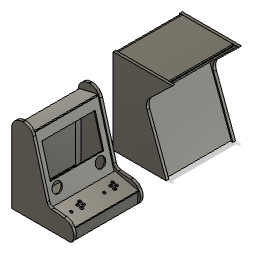
Curvy-Cab (Autodesk Fusion 360 design; units mm, degrees)
Autodesk Fusion 360 part; units mm, degrees
note: some values were not read from the file. Chosen so that the rebuilt part matches the saved one: which bodies a step acts on; which face or edge a step refers to; a side. Set by a fixed rule: which sketch regions a step uses.
sketch "Sketch1" plane through (0, 0, 0) normal (0, 0, 1) x (1, 0, 0)
  line L0 (0, 0) -> (508, 0)
  line L1 (0, 0) -> (0, 1478.2685)
  line L2 (205.4071, 1505.406) -> (336.1627, 1032.1467)
  line L3 (381.7704, 993.9985) -> (500.0828, 983.0939)
  line L4 (561.4783, 808.976) -> (349.2633, 603.2383)
  line L5 (324.7055, 495.0118) -> (508, 0)
  arc A0 (336.1627, 1032.1467) -> (381.7704, 993.9985) centre (386.57, 1046.0736) ccw
  arc A1 (561.4783, 808.976) -> (500.0828, 983.0939) centre (490.7581, 881.9227) ccw
  arc A2 (349.2633, 603.2383) -> (324.7055, 495.0118) centre (419.9835, 530.2916) ccw
  line L6 (100.21, 1579.8589) -> (106.0861, 1579.9393)
  arc A3 (100.21, 1579.8589) -> (0, 1478.2685) centre (101.6, 1478.2685) ccw
  arc A4 (205.4071, 1505.406) -> (106.0861, 1579.9393) centre (107.4762, 1478.3489) ccw
  point P0 (0, 1651)
  dimension "d1" = 508
  dimension "d2" = 1651
  dimension "d48" = 101.6
  dimension "d49" = 101.6
  constraint coincident L0.start L1.start
  constraint horizontal L0
  constraint perpendicular L0 L1
  constraint coincident P0 L1
  constraint tangent L2 A0
  constraint tangent L3 A0
  constraint tangent L3 A1
  constraint tangent L4 A1
  constraint tangent L4 A2
  constraint tangent L5 A2
  constraint tangent L1 A3
  constraint tangent L6 A3
  constraint tangent L2 A4
  constraint tangent L6 A4
  measures "d1" distance of L0.start L0.end
  measures "d2" distance of L0.start P0
  measures "d48" radius of A3
  measures "d49" radius of A4
extrude "Extrude1" add sketch "Sketch1" along normal blind 25.4 makes body 1
copy_body "CopyPasteBodies2" bodies 1 makes body 2
move_body "Move5" bodies 2 to x (1, 0, 0) y (0, 1, 0) z (0, 0, 1) at (0, 0, -635)
sketch "Sketch17" plane through (0, 0, 0) normal (0, 0, 1) x (1, 0, 0)
  line L0 (0, 0) -> (502.8778, 0)
  constraint coincident L0.start origin
  constraint horizontal L0
extrude "Extrude15" add sketch "Sketch17" against normal up to surface (609.6 mm away) thin wall 12.7 on the left separate body open curves L0 makes body 3
extrude "Extrude16" cut 1 faces at (0, 8.4667, -203.2) along direction (1, 0, 0) blind 25.4 on bodies 3 bodies 3
extrude "Extrude17" cut 1 faces at (502.8778, 8.4667, -203.2) along direction (-1, 0, 0) blind 25.4 on bodies 3 bodies 3
sketch "Sketch19" plane through (0, 0, 0) normal (0, 0, -1) x (-1, 0, 0)
  line L0 (-205.4071, 1505.406) -> (-336.1627, 1032.1467)
  arc A0 (-381.7704, 993.9985) -> (-336.1627, 1032.1467) centre (-386.57, 1046.0736) ccw
  line L1 (-381.7704, 993.9985) -> (-500.0828, 983.0939)
  arc A1 (-500.0828, 983.0939) -> (-561.4783, 808.976) centre (-490.7581, 881.9227) ccw
  line L2 (-561.4783, 808.976) -> (-349.2633, 603.2383)
  arc A2 (-324.7055, 495.0118) -> (-349.2633, 603.2383) centre (-419.9835, 530.2916) ccw
  line L3 (-324.7055, 495.0118) -> (-508, 0)
  line L4 (-508, 0) -> (0, 0)
  line L5 (0, 0) -> (0, 1478.2685)
  arc A3 (0, 1478.2685) -> (-100.21, 1579.8589) centre (-101.6, 1478.2685) ccw
  line L6 (-100.21, 1579.8589) -> (-106.0861, 1579.9393)
  arc A4 (-106.0861, 1579.9393) -> (-205.4071, 1505.406) centre (-107.4762, 1478.3489) ccw
  line L7 (0, 0) -> (0, 1478.2685)
  constraint coincident L4.end L5.start
  constraint coincident L5.end A3.start
extrude "Extrude18" add sketch "Sketch19" along normal up to surface (609.6 mm away) thin wall 12.7 on the left separate body open curves L7 makes body 4
move_body "Move6" bodies 4 to x (1, 0, 0) y (0, 1, 0) z (0, 0, 1) at (12.7, 0, 0)
sketch "Sketch20" plane through (0, 0, 0) normal (0, 0, -1) x (-1, 0, 0)
  line L0 (-205.4071, 1505.406) -> (-336.1627, 1032.1467)
  arc A0 (-381.7704, 993.9985) -> (-336.1627, 1032.1467) centre (-386.57, 1046.0736) ccw
  line L1 (-381.7704, 993.9985) -> (-500.0828, 983.0939)
  arc A1 (-500.0828, 983.0939) -> (-561.4783, 808.976) centre (-490.7581, 881.9227) ccw
  line L2 (-561.4783, 808.976) -> (-349.2633, 603.2383)
  arc A2 (-324.7055, 495.0118) -> (-349.2633, 603.2383) centre (-419.9835, 530.2916) ccw
  line L3 (-324.7055, 495.0118) -> (-508, 0)
  line L4 (-508, 0) -> (0, 0)
  line L5 (0, 0) -> (0, 1478.2685)
  arc A3 (0, 1478.2685) -> (-100.21, 1579.8589) centre (-101.6, 1478.2685) ccw
  line L6 (-100.21, 1579.8589) -> (-106.0861, 1579.9393)
  arc A4 (-106.0861, 1579.9393) -> (-205.4071, 1505.406) centre (-107.4762, 1478.3489) ccw
  line L7 (-508, 0) -> (-289.0482, 591.3093)
  constraint coincident L3.end L4.start
  constraint parallel L3 L7
extrude "Extrude19" add sketch "Sketch20" along normal up to surface (609.6 mm away) thin wall 12.7 on the left separate body open curves L7 makes body 5
move_body "Move7" bodies 5 to x (1, 0, 0) y (0, 1, 0) z (0, 0, 1) at (-23.8195, -8.82, 0)
extrude "Extrude20" cut 1 faces at (492.1203, -5.88, -203.2) along direction (-0.347242, 0.937775, 0) blind 12.7 on bodies 5 bodies 5
sketch "Sketch21" plane through (0, 0, 0) normal (0, 0, -1) x (-1, 0, 0)
  line L0 (-205.4071, 1505.406) -> (-336.1627, 1032.1467)
  arc A0 (-381.7704, 993.9985) -> (-336.1627, 1032.1467) centre (-386.57, 1046.0736) ccw
  line L1 (-381.7704, 993.9985) -> (-500.0828, 983.0939)
  arc A1 (-500.0828, 983.0939) -> (-561.4783, 808.976) centre (-490.7581, 881.9227) ccw
  line L2 (-561.4783, 808.976) -> (-349.2633, 603.2383)
  arc A2 (-324.7055, 495.0118) -> (-349.2633, 603.2383) centre (-419.9835, 530.2916) ccw
  line L3 (-324.7055, 495.0118) -> (-508, 0)
  line L4 (-508, 0) -> (0, 0)
  line L5 (0, 0) -> (0, 1478.2685)
  arc A3 (0, 1478.2685) -> (-100.21, 1579.8589) centre (-101.6, 1478.2685) ccw
  line L6 (-100.21, 1579.8589) -> (-106.0861, 1579.9393)
  arc A4 (-106.0861, 1579.9393) -> (-205.4071, 1505.406) centre (-107.4762, 1478.3489) ccw
  line L7 (-284.5357, 560.5229) -> (-561.4783, 835.6804)
extrude "Extrude21" add sketch "Sketch21" along normal up to surface (609.6 mm away) thin wall 12.7 on the left separate body open curves L7 makes body 6
sketch "Sketch22" plane through (0, 0, 0) normal (0, 0, -1) x (-1, 0, 0)
  line L0 (-205.4071, 1505.406) -> (-336.1627, 1032.1467)
  arc A0 (-381.7704, 993.9985) -> (-336.1627, 1032.1467) centre (-386.57, 1046.0736) ccw
  line L1 (-381.7704, 993.9985) -> (-500.0828, 983.0939)
  arc A1 (-500.0828, 983.0939) -> (-561.4783, 808.976) centre (-490.7581, 881.9227) ccw
  line L2 (-561.4783, 808.976) -> (-349.2633, 603.2383)
  arc A2 (-324.7055, 495.0118) -> (-349.2633, 603.2383) centre (-419.9835, 530.2916) ccw
  line L3 (-324.7055, 495.0118) -> (-508, 0)
  line L4 (-508, 0) -> (0, 0)
  line L5 (0, 0) -> (0, 1478.2685)
  arc A3 (0, 1478.2685) -> (-100.21, 1579.8589) centre (-101.6, 1478.2685) ccw
  line L6 (-100.21, 1579.8589) -> (-106.0861, 1579.9393)
  arc A4 (-106.0861, 1579.9393) -> (-205.4071, 1505.406) centre (-107.4762, 1478.3489) ccw
  line L7 (-551.3631, 829.4223) -> (-558.7598, 935.9349)
extrude "Extrude22" add sketch "Sketch22" along normal up to surface (609.6 mm away) thin wall 12.7 on the left separate body open curves L7 makes body 7
move_face "MoveFace1" by (12.6695, -0.8798, 0) 1 faces at (566.4981, 864.0467, -203.2) on bodies 7
move_body "Move8" bodies 7 to x (1, 0, 0) y (0, 1, 0) z (0, 0, 1) at (-6.3347, 0.4399, 0)
extrude "Extrude23" cut 1 faces at (569.3177, 935.2017, -203.2) along direction (-0.069278, -0.997597, 0) blind 6.35 on bodies 7 bodies 7
move_body "Move9" bodies 6 to x (1, 0, 0) y (0, 1, 0) z (0, 0, 1) at (-4.4756, 4.5046, 0)
move_body "Move10" bodies 7 to x (1, 0, 0) y (0, 1, 0) z (0, 0, 1) at (-6.3347, 0.4399, 0)
sketch "Sketch23" plane through (0, 0, 0) normal (0, 0, -1) x (-1, 0, 0)
  line L0 (-205.4071, 1505.406) -> (-336.1627, 1032.1467)
  arc A0 (-381.7704, 993.9985) -> (-336.1627, 1032.1467) centre (-386.57, 1046.0736) ccw
  line L1 (-381.7704, 993.9985) -> (-500.0828, 983.0939)
  arc A1 (-500.0828, 983.0939) -> (-561.4783, 808.976) centre (-490.7581, 881.9227) ccw
  line L2 (-561.4783, 808.976) -> (-349.2633, 603.2383)
  arc A2 (-324.7055, 495.0118) -> (-349.2633, 603.2383) centre (-419.9835, 530.2916) ccw
  line L3 (-324.7055, 495.0118) -> (-508, 0)
  line L4 (-508, 0) -> (0, 0)
  line L5 (0, 0) -> (0, 1478.2685)
  arc A3 (0, 1478.2685) -> (-100.21, 1579.8589) centre (-101.6, 1478.2685) ccw
  line L6 (-100.21, 1579.8589) -> (-106.0861, 1579.9393)
  arc A4 (-106.0861, 1579.9393) -> (-205.4071, 1505.406) centre (-107.4762, 1478.3489) ccw
  line L7 (-559.5268, 925.2519) -> (-297.9673, 983.8984)
extrude "Extrude24" add sketch "Sketch23" along normal up to surface (609.6 mm away) thin wall 12.7 on the left separate body open curves L7 makes body 8
move_body "Move11" bodies 8 to x (1, 0, 0) y (0, 1, 0) z (0, 0, 1) at (-1.3893, -6.1962, 0)
extrude "Extrude25" cut 1 faces at (298.4304, 985.9638, -406.4) along direction (0.975773, -0.218786, 0) blind 50.8 on bodies 8 bodies 8
sketch "Sketch24" plane through (0, 0, 0) normal (0, 0, -1) x (-1, 0, 0)
  line L0 (-205.4071, 1505.406) -> (-336.1627, 1032.1467)
  arc A0 (-381.7704, 993.9985) -> (-336.1627, 1032.1467) centre (-386.57, 1046.0736) ccw
  line L1 (-381.7704, 993.9985) -> (-500.0828, 983.0939)
  arc A1 (-500.0828, 983.0939) -> (-561.4783, 808.976) centre (-490.7581, 881.9227) ccw
  line L2 (-561.4783, 808.976) -> (-349.2633, 603.2383)
  arc A2 (-324.7055, 495.0118) -> (-349.2633, 603.2383) centre (-419.9835, 530.2916) ccw
  line L3 (-324.7055, 495.0118) -> (-508, 0)
  line L4 (-508, 0) -> (0, 0)
  line L5 (0, 0) -> (0, 1478.2685)
  arc A3 (0, 1478.2685) -> (-100.21, 1579.8589) centre (-101.6, 1478.2685) ccw
  line L6 (-100.21, 1579.8589) -> (-106.0861, 1579.9393)
  arc A4 (-106.0861, 1579.9393) -> (-205.4071, 1505.406) centre (-107.4762, 1478.3489) ccw
  line L7 (-336.1627, 1032.1467) -> (-205.4071, 1505.406)
  constraint coincident L0.end A0.end
  constraint coincident L0.start A4.end
extrude "Extrude26" add sketch "Sketch24" along normal up to surface (609.6 mm away) thin wall 12.7 on the left separate body open curves L7 makes body 9
move_body "Move12" bodies 9 to x (1, 0, 0) y (0, 1, 0) z (0, 0, 1) at (-24.4827, -6.7643, 0)
move_body "Move13" bodies 9 to x (1, 0, 0) y (0, 1, 0) z (0, 0, 1) at (73.4482, 20.2928, 0)
extrude "Extrude27" add 1 faces at (393.2891, 1047.93, -203.2) along direction (0.26631, -0.963887, 0) blind 50.8 on bodies 9 bodies 9
move_body "Move14" bodies 9 to x (1, 0, 0) y (0, 1, 0) z (0, 0, 1) at (152.4, 0, 0)
move_body "Move15" bodies 9 to x (1, 0, 0) y (0, 1, 0) z (0, 0, 1) at (97.931, 27.0571, 0)
extrude "Extrude28" add 1 faces at (657.1486, 1026.0216, -203.2) along direction (0.26631, -0.963887, 0) blind 25.4 on bodies 9 bodies 9
move_body "Move16" bodies 9 to x (1, 0, 0) y (0, 1, 0) z (0, 0, 1) at (-318.2756, -87.9356, 0)
move_body "Move17" bodies 9 to x (1, 0, 0) y (0, 1, 0) z (0, 0, 1) at (4.8965, 1.3529, 0)
move_body "Move18" bodies 7 to x (1, 0, 0) y (0, 1, 0) z (0, 0, 1) at (76.0169, -5.279, 0)
extrude "Extrude29" cut 1 faces at (638.56, 924.0279, -203.2) along direction (-0.069278, -0.997597, 0) blind 12.7 on bodies 7 bodies 7
move_body "Move19" bodies 8 to x (1, 0, 0) y (0, 1, 0) z (0, 0, 1) at (38.9002, 173.4924, 0)
extrude "Extrude30" add 1 faces at (598.8901, 1100.8096, -203.2) along direction (0.975773, -0.218786, 0) blind 12.7 on bodies 8 bodies 8
extrude "Extrude31" cut 1 faces at (642.0751, 852.433, -406.4) along direction (-0.997597, 0.069278, 0) blind 12.7 on bodies 7 bodies 7
move_body "Move20" bodies 7 to x (1, 0, 0) y (0, 1, 0) z (0, 0, 1) at (-63.3474, 4.3991, 0)
move_body "Move21" bodies 8 to x (1, 0, 0) y (0, 1, 0) z (0, 0, 1) at (-38.9002, -173.4924, 0)
sketch "Sketch25" plane through (564.6168, 155.9965, 0) normal (0.963887, 0.26631, 0) x (0, 0, -1)
  line L0 (609.6, 788.5641) -> (609.6, 1355.7543)
  line L1 (609.6, 1355.7543) -> (0, 1355.7543)
  line L2 (0, 1355.7543) -> (0, 788.5641)
  line L3 (0, 788.5641) -> (609.6, 788.5641)
  line L4 (50.8, 1279.5543) -> (558.8, 1279.5543)
  line L5 (558.8, 1279.5543) -> (558.8, 974.7543)
  line L6 (558.8, 974.7543) -> (50.8, 974.7543)
  line L7 (50.8, 974.7543) -> (50.8, 1279.5543)
  dimension "d94" = 508
  dimension "d95" = 304.8
  constraint horizontal L4
  constraint vertical L5
  constraint horizontal L6
  constraint vertical L7
  measures "d94" distance of L4.start L4.end
  measures "d95" distance of L4.start L6.end
extrude "Extrude32" cut sketch "Sketch25" against normal blind 12.7 contours L4 L5 L6 L7 bodies 9
sketch "Sketch26" plane through (0, 0, 0) normal (0, 0, -1) x (-1, 0, 0)
  line L0 (-205.4071, 1505.406) -> (-336.1627, 1032.1467)
  arc A0 (-381.7704, 993.9985) -> (-336.1627, 1032.1467) centre (-386.57, 1046.0736) ccw
  line L1 (-381.7704, 993.9985) -> (-500.0828, 983.0939)
  arc A1 (-500.0828, 983.0939) -> (-561.4783, 808.976) centre (-490.7581, 881.9227) ccw
  line L2 (-561.4783, 808.976) -> (-349.2633, 603.2383)
  arc A2 (-324.7055, 495.0118) -> (-349.2633, 603.2383) centre (-419.9835, 530.2916) ccw
  line L3 (-324.7055, 495.0118) -> (-508, 0)
  line L4 (-508, 0) -> (0, 0)
  line L5 (0, 0) -> (0, 1478.2685)
  arc A3 (0, 1478.2685) -> (-100.21, 1579.8589) centre (-101.6, 1478.2685) ccw
  line L6 (-100.21, 1579.8589) -> (-106.0861, 1579.9393)
  arc A4 (-106.0861, 1579.9393) -> (-205.4071, 1505.406) centre (-107.4762, 1478.3489) ccw
  line L7 (-200.4269, 1464.4958) -> (-22.4744, 1480.1356)
extrude "Extrude33" add sketch "Sketch26" along normal up to surface (609.6 mm away) thin wall 12.7 on the left separate body open curves L7 makes body 10
move_body "Move22" bodies 10 to x (1, 0, 0) y (0, 1, 0) z (0, 0, 1) at (15.5664, 177.1173, 0)
extrude "Extrude34" add 1 faces at (38.7821, 1665.687, -203.2) along direction (-0.99616, 0.08755, 0) blind 12.7 on bodies 10 bodies 10
move_body "Move23" bodies 10 to x (1, 0, 0) y (0, 1, 0) z (0, 0, 1) at (-15.5664, -177.1173, 0)
move_body "Move24" bodies 10 to x (1, 0, 0) y (0, 1, 0) z (0, 0, 1) at (15.5664, 177.1173, 0)
extrude "Extrude35" cut 1 faces at (21.1667, 1478.2685, -203.2) along direction (0, -1, 0) blind 25.4 on bodies 4 bodies 4
move_body "Move25" bodies 10 to x (0.996195, 0.087156, 0) y (-0.087156, 0.996195, 0) z (0, 0, 1) at (145.2393, 17.8668, 0)
move_body "Move26" bodies 9 to x (1, 0, 0) y (0, 1, 0) z (0, 0, 1) at (122.4137, 33.8214, 0)
extrude "Extrude36" add 1 faces at (321.8991, 1495.485, -406.4) along direction (-0.26631, 0.963887, 0) blind 25.4 on bodies 9 bodies 9
move_body "Move27" bodies 9 to x (1, 0, 0) y (0, 1, 0) z (0, 0, 1) at (-122.4137, -33.8214, 0)
extrude "Extrude37" cut 1 faces at (21.1667, 1452.8685, -203.2) along direction (0, -1, 0) blind 25.4 on bodies 4 bodies 4
move_body "Move28" bodies 10 to x (0.951057, 0.309017, 0) y (-0.309017, 0.951057, 0) z (0, 0, 1) at (503.5292, -166.7296, 0)
move_body "Move29" bodies 10 to x (1, 0, 0) y (0, 1, 0) z (0, 0, 1) at (1.5679, -4.832, 0)
sketch "Sketch27" plane through (12.7, 0, 0) normal (-1, 0, 0) x (0, 0, 1)
  line L0 (0, 1427.4685) -> (-609.6, 1427.4685)
  line L1 (-609.6, 1427.4685) -> (-609.6, 0)
  line L2 (-609.6, 0) -> (0, 0)
  line L3 (0, 0) -> (0, 1427.4685)
sketch "Sketch28" plane through (0, 0, 0) normal (1, 0, 0) x (0, 0, -1)
  line L0 (-739.8755, 1382.7471) -> (-238.2255, 1382.7471)
  line L1 (-238.2255, 1382.7471) -> (-238.2255, 271.4971)
  line L2 (-238.2255, 271.4971) -> (-739.8755, 271.4971)
  line L3 (-739.8755, 271.4971) -> (-739.8755, 1382.7471)
  dimension "d113" = 501.65
  dimension "d114" = 1111.25
  constraint horizontal L0
  constraint vertical L1
  constraint horizontal L2
  constraint vertical L3
  measures "d113" distance of L0.start L0.end
  measures "d114" distance of L0.start L2.end
sketch "Sketch29" plane through (12.7, 0, 0) normal (-1, 0, 0) x (0, 0, 1)
  line L0 (0, 1427.4685) -> (-609.6, 1427.4685)
  line L1 (-609.6, 1427.4685) -> (-609.6, 0)
  line L2 (-609.6, 0) -> (0, 0)
  line L3 (0, 0) -> (0, 1427.4685)
  line L4 (-87.375, 145.627) -> (-61.975, 145.627)
  line L5 (-61.975, 145.627) -> (-61.975, 97.367)
  line L6 (-61.975, 97.367) -> (-87.375, 97.367)
  line L7 (-87.375, 97.367) -> (-87.375, 145.627)
  dimension "d117" = 25.4
  dimension "d118" = 48.26
  constraint horizontal L4
  constraint vertical L5
  constraint horizontal L6
  constraint vertical L7
  measures "d117" distance of L4.start L4.end
  measures "d118" distance of L4.start L6.end
extrude "Extrude40" cut sketch "Sketch29" against normal blind 12.7 contours L4 L5 L6 L7 bodies 4
sketch "Sketch30" plane through (564.6168, 155.9965, 0) normal (0.963887, 0.26631, 0) x (0, 0, -1)
  line L0 (558.8, 1279.5543) -> (558.8, 974.7543)
  line L1 (558.8, 974.7543) -> (50.8, 974.7543)
  line L2 (50.8, 974.7543) -> (50.8, 1279.5543)
  line L3 (50.8, 1279.5543) -> (558.8, 1279.5543)
  line L4 (609.6, 788.5641) -> (609.6, 1381.1543)
  line L5 (609.6, 1381.1543) -> (0, 1381.1543)
  line L6 (0, 1381.1543) -> (0, 788.5641)
  line L7 (0, 788.5641) -> (609.6, 788.5641)
  circle A0 centre (98.425, 908.9287) radius 47.625
  circle A1 centre (511.175, 908.9287) radius 47.625
  dimension "d121" = 95.25
  dimension "d122" = 95.25
  constraint tangent L2 A0
  constraint tangent L0 A1
  measures "d121" diameter of A0
  measures "d122" diameter of A1
extrude "Extrude41" cut sketch "Sketch30" against normal blind 12.7 contours A0 | A1 bodies 9
sketch "Sketch31" plane through (225.7006, 1006.6096, 0) normal (0.218786, 0.975773, 0) x (0, 0, -1)
  line L0 (609.6, -126.2847) -> (0, -126.2847)
  line L1 (0, -126.2847) -> (0, -356.2385)
  line L2 (0, -356.2385) -> (609.6, -356.2385)
  line L3 (609.6, -356.2385) -> (609.6, -126.2847)
  circle A0 centre (171.8305, -213.1243) radius 14.2875
  circle A1 centre (204.8505, -198.1383) radius 14.2875
  circle A2 centre (204.8505, -234.2345) radius 14.2875
  circle A3 centre (171.8305, -249.5498) radius 14.2875
  circle A4 centre (88.2645, -234.2345) radius 12.7
  circle A5 centre (486.728, -213.1243) radius 14.2875
  circle A6 centre (519.748, -198.1383) radius 14.2875
  circle A7 centre (519.748, -234.2345) radius 14.2875
  circle A8 centre (486.728, -249.5498) radius 14.2875
  circle A9 centre (403.162, -234.2345) radius 12.7
extrude "Extrude42" cut sketch "Sketch31" against normal blind 12.7 contours A0 | A1 | A2 | A3 | A4 | A5 | A6 | A7 | A8 | A9 bodies 8
move_body "Move30" bodies 9 10 to x (1, 0, 0) y (0, 1, 0) z (0, 0, 1) at (0, 50.8, 0)
move_body "Move31" bodies 10 to x (1, 0, 0) y (0, 1, 0) z (0, 0, 1) at (0, 50.8, 0)
move_body "Move32" bodies 4 to x (1, 0, 0) y (0, 1, 0) z (0, 0, 1) at (-76.2, 0, 0)
extrude "Extrude43" add 1 faces at (-55.0333, 1427.4685, -203.2) along direction (0, 1, 0) blind 50.8 on bodies 4 bodies 4
move_body "Move33" bodies 4 to x (1, 0, 0) y (0, 1, 0) z (0, 0, 1) at (76.2, 0, 0)
move_body "Move34" bodies 10 to x (1, 0, 0) y (0, 1, 0) z (0, 0, 1) at (15.6789, -48.3199, 0)
move_body "Move35" bodies 10 to x (1, 0, 0) y (0, 1, 0) z (0, 0, 1) at (-24.1599, -7.8395, 0)
move_body "Move36" bodies 9 to x (1, 0, 0) y (0, 1, 0) z (0, 0, 1) at (171.3792, 47.3499, 0)
extrude "Extrude44" cut 1 faces at (364.1003, 1584.2963, -406.4) along direction (0.26631, -0.963887, 0) blind 12.7 on bodies 9 bodies 9
move_body "Move37" bodies 9 to x (1, 0, 0) y (0, 1, 0) z (0, 0, 1) at (-183.6206, -50.7321, 0)
move_body "Move38" bodies 10 to x (0.996195, -0.087156, 0) y (0.087156, 0.996195, 0) z (0, 0, 1) at (-130.9638, 9.4206, 0)
move_body "Move39" bodies 10 to x (1, 0, 0) y (0, 1, 0) z (0, 0, 1) at (-62.7436, 272.2639, 0)
extrude "Extrude45" cut 1 faces at (-62.6928, 1756.1359, -203.2) along direction (0.974459, 0.224565, 0) blind 12.7 on bodies 10 bodies 10
move_body "Move40" bodies 10 to x (1, 0, 0) y (0, 1, 0) z (0, 0, 1) at (62.7436, -272.2639, 0)
sketch "Sketch32" plane through (0, 0, 25.4) normal (0, 0, 1) x (1, 0, 0)
  line L0 (336.1627, 1032.1467) -> (205.4071, 1505.406)
  arc A0 (205.4071, 1505.406) -> (106.0861, 1579.9393) centre (107.4762, 1478.3489) ccw
  line L1 (106.0861, 1579.9393) -> (100.21, 1579.8589)
  arc A1 (100.21, 1579.8589) -> (0, 1478.2685) centre (101.6, 1478.2685) ccw
  line L2 (0, 1478.2685) -> (0, 0)
  line L3 (0, 0) -> (508, 0)
  line L4 (508, 0) -> (324.7055, 495.0118)
  arc A2 (349.2633, 603.2383) -> (324.7055, 495.0118) centre (419.9835, 530.2916) ccw
  line L5 (349.2633, 603.2383) -> (561.4783, 808.976)
  arc A3 (561.4783, 808.976) -> (500.0828, 983.0939) centre (490.7581, 881.9227) ccw
  line L6 (500.0828, 983.0939) -> (381.7704, 993.9985)
  arc A4 (336.1627, 1032.1467) -> (381.7704, 993.9985) centre (386.57, 1046.0736) ccw
  line L7 (0, 0) -> (0, 812.8)
  line L8 (0, 812.8) -> (565.2203, 812.8)
  dimension "d133" = 812.8
  constraint coincident L2.end L3.start
  constraint perpendicular L3 L7
  constraint coincident A3 L8.end
  constraint perpendicular L2 L8
  measures "d133" distance of L2.end L7.end
split "Split1" by curves path "Sketch32" along L7 L8 bodies 1 makes body 11 at (112.0542, 1107.7384, 0)
sketch "Sketch33" plane through (0, 0, -635) normal (0, 0, -1) x (-1, 0, 0)
  line L0 (-205.4071, 1505.406) -> (-336.1627, 1032.1467)
  arc A0 (-381.7704, 993.9985) -> (-336.1627, 1032.1467) centre (-386.57, 1046.0736) ccw
  line L1 (-381.7704, 993.9985) -> (-500.0828, 983.0939)
  arc A1 (-500.0828, 983.0939) -> (-561.4783, 808.976) centre (-490.7581, 881.9227) ccw
  line L2 (-561.4783, 808.976) -> (-349.2633, 603.2383)
  arc A2 (-324.7055, 495.0118) -> (-349.2633, 603.2383) centre (-419.9835, 530.2916) ccw
  line L3 (-324.7055, 495.0118) -> (-508, 0)
  line L4 (-508, 0) -> (0, 0)
  line L5 (0, 0) -> (0, 1478.2685)
  arc A3 (0, 1478.2685) -> (-100.21, 1579.8589) centre (-101.6, 1478.2685) ccw
  line L6 (-100.21, 1579.8589) -> (-106.0861, 1579.9393)
  arc A4 (-106.0861, 1579.9393) -> (-205.4071, 1505.406) centre (-107.4762, 1478.3489) ccw
  line L7 (0, 0) -> (0, 812.8)
  line L8 (0, 812.8) -> (-565.2203, 812.8)
  dimension "d134" = 812.8
  constraint coincident L4.end L5.start
  constraint perpendicular L4 L7
  constraint coincident A1 L8.end
  constraint perpendicular L7 L8
  measures "d134" distance of L4.end L7.end
split "Split2" by curves path "Sketch33" along L7 L8 bodies 2 makes body 12 at (112.0542, 1107.7384, -635)
move_body "Move41" bodies 6 to x (1, 0, 0) y (0, 1, 0) z (0, 0, 1) at (53.707, -54.0555, 0)
extrude "Extrude46" cut 1 faces at (616.6772, 780.1234, -203.2) along direction (-0.709389, -0.704817, 0) blind 25.4 on bodies 6 bodies 6
extrude "Extrude47" cut 1 faces at (598.6587, 762.221, -203.2) along direction (-0.709389, -0.704817, 0) blind 12.7 on bodies 6 bodies 6
move_body "Move42" bodies 6 to x (1, 0, 0) y (0, 1, 0) z (0, 0, 1) at (-53.707, 54.0555, 0)
sketch "Sketch34" plane through (0, 0, 0) normal (0, 0, -1) x (-1, 0, 0)
  line L0 (-565.2203, 812.8) -> (0, 812.8)
  line L1 (0, 812.8) -> (0, 1478.2685)
  arc A0 (0, 1478.2685) -> (-100.21, 1579.8589) centre (-101.6, 1478.2685) ccw
  line L2 (-100.21, 1579.8589) -> (-106.0861, 1579.9393)
  arc A1 (-106.0861, 1579.9393) -> (-205.4071, 1505.406) centre (-107.4762, 1478.3489) ccw
  line L3 (-205.4071, 1505.406) -> (-336.1627, 1032.1467)
  arc A2 (-381.7704, 993.9985) -> (-336.1627, 1032.1467) centre (-386.57, 1046.0736) ccw
  line L4 (-381.7704, 993.9985) -> (-500.0828, 983.0939)
  arc A3 (-500.0828, 983.0939) -> (-565.2203, 812.8) centre (-490.7581, 881.9227) ccw
sketch "Sketch35" plane through (0, 0, 0) normal (0, 0, -1) x (-1, 0, 0)
sketch "Sketch36" plane through (0, 0, 0) normal (0, 0, -1) x (-1, 0, 0)
  line L0 (-0.1321, 812.1031) -> (-562.8374, 812.1031)
  constraint horizontal L0
extrude "Extrude48" add sketch "Sketch36" along normal up to surface (609.6 mm away) thin wall 12.7 on the left separate body open curves L0 makes body 13
move_body "Move43" bodies 13 to x (1, 0, 0) y (0, 1, 0) z (0, 0, 1) at (1117.6, 12.7, 0)
extrude "Extrude49" cut 1 faces at (1117.7321, 816.3364, -203.2) along direction (1, 0, 0) blind 25.4 on bodies 13 bodies 13
move_body "Move44" bodies 13 to x (1, 0, 0) y (0, 1, 0) z (0, 0, 1) at (-1117.6, 0, 0)
sketch "Sketch37" plane through (12.7, 0, 0) normal (-1, 0, 0) x (0, 0, 1)
  line L0 (-61.975, 145.627) -> (-61.975, 97.367)
  line L1 (-61.975, 97.367) -> (-87.375, 97.367)
  line L2 (-87.375, 97.367) -> (-87.375, 145.627)
  line L3 (-87.375, 145.627) -> (-61.975, 145.627)
  line L4 (-609.6, 1478.2685) -> (-609.6, 0)
  line L5 (-609.6, 0) -> (0, 0)
  line L6 (0, 0) -> (0, 1478.2685)
  line L7 (0, 1478.2685) -> (-609.6, 1478.2685)
sketch "Sketch38" plane through (12.7, 0, 0) normal (-1, 0, 0) x (0, 0, 1)
  line L0 (0, 812.8) -> (-609.6, 812.8)
  dimension "d145" = 609.6
  measures "d145" distance of L0.start L0.end
split "Split3" by curves path "Sketch38" along L0 bodies 4 makes body 14 at (25.4, 1034.6228, -203.2)
move_body "Move45" bodies 13 to x (1, 0, 0) y (0, 1, 0) z (0, 0, 1) at (660.4, 0, 0)
extrude "Extrude50" cut 1 faces at (1223.2374, 816.3364, -203.2) along direction (-1, 0, 0) blind 12.7 on bodies 13 bodies 13
move_body "Move46" bodies 13 to x (1, 0, 0) y (0, 1, 0) z (0, 0, 1) at (-660.4, 0, 0)
move_body "Move47" bodies 10 9 7 12 13 14 11 8 to x (1, 0, 0) y (0, 1, 0) z (0, 0, 1) at (0, 355.6, 0)
move_body "Move48" bodies 14 9 7 12 10 13 11 8 to x (1, 0, 0) y (0, 1, 0) z (0, 0, 1) at (0, -1168.4, 1092.2)
move_body "Move49" bodies 7 to x (1, 0, 0) y (0, 1, 0) z (0, 0, 1) at (101.3559, -7.0386, 0)
extrude "Extrude51" add 1 faces at (661.1653, 8.9972, 889) along direction (-0.069278, -0.997597, 0) blind 12.7 on bodies 7 bodies 7
move_body "Move50" bodies 7 to x (1, 0, 0) y (0, 1, 0) z (0, 0, 1) at (-101.3559, 7.0386, 0)
move_body "Move51" bodies 7 to x (1, 0, 0) y (0, 1, 0) z (0, 0, 1) at (101.3559, -7.0386, 0)
extrude "Extrude52" add 1 faces at (660.2855, -3.6723, 889) along direction (-0.069278, -0.997597, 0) blind 2.54 on bodies 7 bodies 7
move_body "Move52" bodies 7 to x (1, 0, 0) y (0, 1, 0) z (0, 0, 1) at (-101.3559, 7.0386, 0)
sketch "Sketch39" plane through (0, 0, 0) normal (0, 0, -1) x (-1, 0, 0)
  line L0 (0, 812.8) -> (-565.2203, 812.8)
  arc A0 (-565.2203, 812.8) -> (-561.4783, 808.976) centre (-490.7581, 881.9227) ccw
  line L1 (-561.4783, 808.976) -> (-349.2633, 603.2383)
  arc A1 (-324.7055, 495.0118) -> (-349.2633, 603.2383) centre (-419.9835, 530.2916) ccw
  line L2 (-324.7055, 495.0118) -> (-508, 0)
  line L3 (-508, 0) -> (0, 0)
  line L4 (0, 0) -> (0, 812.8)
  line L5 (-25.4507, 812.8) -> (-509.0368, 812.8)
  constraint coincident L0 L5.start
  constraint coincident L0 L5.end
extrude "Extrude53" add sketch "Sketch39" along normal up to surface (609.6 mm away) thin wall 12.7 on the left separate body open curves L5 makes body 15
sketch "Sketch40" plane through (12.7, 0, 0) normal (-1, 0, 0) x (0, 0, 1)
  line L0 (-558.8, 723.9) -> (-50.8, 723.9)
  line L1 (-50.8, 723.9) -> (-50.8, 215.9)
  line L2 (-50.8, 215.9) -> (-558.8, 215.9)
  line L3 (-558.8, 215.9) -> (-558.8, 723.9)
  line L4 (0, 800.1) -> (-609.6, 800.1)
  dimension "d156" = 508
  dimension "d157" = 508
  constraint horizontal L0
  constraint vertical L1
  constraint horizontal L2
  constraint vertical L3
  measures "d156" distance of L0.start L0.end
  measures "d157" distance of L0.start L2.end
extrude "Extrude54" cut sketch "Sketch40" against normal blind 12.7 bodies 4
sketch "Sketch41" plane through (12.7, 0, 0) normal (-1, 0, 0) x (0, 0, 1)
  line L0 (482.6, 0) -> (1092.2, 0)
  line L1 (1092.2, 0) -> (1092.2, 665.4685)
  line L2 (1092.2, 665.4685) -> (482.6, 665.4685)
  line L3 (482.6, 665.4685) -> (482.6, 0)
  line L4 (533.4, 589.2685) -> (1041.4, 589.2685)
  line L5 (1041.4, 589.2685) -> (1041.4, 81.2685)
  line L6 (1041.4, 81.2685) -> (533.4, 81.2685)
  line L7 (533.4, 81.2685) -> (533.4, 589.2685)
  dimension "d160" = 508
  dimension "d161" = 508
  constraint horizontal L4
  constraint vertical L5
  constraint horizontal L6
  constraint vertical L7
  measures "d160" distance of L4.start L4.end
  measures "d161" distance of L4.start L6.end
extrude "Extrude55" cut sketch "Sketch41" against normal blind 12.7 contours L4 L5 L6 L7 bodies 14
sketch "Sketch42" plane through (0, 0, 0) normal (1, 0, 0) x (0, 0, -1)
  line L0 (1070.5868, 803.295) -> (1572.2368, 803.295)
  line L1 (1572.2368, 803.295) -> (1572.2368, 301.645)
  line L2 (1572.2368, 301.645) -> (1070.5868, 301.645)
  line L3 (1070.5868, 301.645) -> (1070.5868, 803.295)
  dimension "d164" = 501.65
  dimension "d165" = 501.65
  constraint horizontal L0
  constraint vertical L1
  constraint horizontal L2
  constraint vertical L3
  measures "d164" distance of L0.start L0.end
  measures "d165" distance of L0.start L2.end
extrude "Extrude56" add sketch "Sketch42" along normal blind 12.7 separate body makes body 16
copy_body "CopyPasteBodies3" bodies 16 makes body 17
move_body "Move53" bodies 17 to x (1, 0, 0) y (0, 1, 0) z (0, 0, 1) at (0, 0, -558.8)
move_body "Move54" bodies 11 14 8 12 7 10 13 9 to x (1, 0, 0) y (0, 1, 0) z (0, 0, 1) at (5.6309, 814.3665, -1092.2)
move_body "Move55" bodies 16 to x (1, 0, 0) y (0, 1, 0) z (0, 0, 1) at (12.7, -82.55, 1016)
move_body "Move56" bodies 17 to x (1, 0, 0) y (0, 1, 0) z (0, 0, 1) at (12.7, 609.6, 1574.8)
move_body "Move57" bodies 17 to x (1, 0, 0) y (0, 1, 0) z (0, 0, 1) at (6.35, -12.7, 0)
move_body "Move58" bodies 10 9 7 13 12 8 11 14 17 to x (1, 0, 0) y (0, 1, 0) z (0, 0, 1) at (-6.35, 0, 0)
move_body "Move59" bodies 17 11 14 13 7 8 10 12 9 to x (1, 0, 0) y (0, 1, 0) z (0, 0, 1) at (0, -812.8, 965.2)
copy_body "Body->Comp1" bodies 13 removing the originals makes body 18 in component "UpperShelf"
copy_body "Body->Comp2" bodies 3 removing the originals makes body 19 in component "Bottom"
copy_body "Body->Comp3" bodies 7 removing the originals makes body 20 in component "FrontConsole"
copy_body "Body->Comp4" bodies 2 removing the originals makes body 21 in component "SideR Bottom"
copy_body "Body->Comp5" bodies 17 removing the originals makes body 22 in component "BottomDoor"
copy_body "Body->Comp6" bodies 4 removing the originals makes body 23 in component "Back Bottom"
copy_body "Body->Comp7" bodies 11 removing the originals makes body 24 in component "SideLTop"
copy_body "Body->Comp8" bodies 1 removing the originals makes body 25 in component "SideLBottom"
copy_body "Body->Comp9" bodies 5 removing the originals makes body 26 in component "FrontLower"
copy_body "Body->Comp10" bodies 12 removing the originals makes body 27 in component "SideR Top"
copy_body "Body->Comp11" bodies 9 removing the originals makes body 28 in component "Screen"
copy_body "Body->Comp12" bodies 8 removing the originals makes body 29 in component "Console"
copy_body "Body->Comp13" bodies 14 removing the originals makes body 30 in component "Back Top"
copy_body "Body->Comp14" bodies 15 removing the originals makes body 31 in component "LowerShelf"
copy_body "Body->Comp15" bodies 10 removing the originals makes body 32 in component "Top"
copy_body "Body->Comp16" bodies 6 removing the originals makes body 33 in component "FrontUpper"
copy_body "Body->Comp17" bodies 16 removing the originals makes body 34 in component "TopDoor"
copy_body "CopyPasteBodies1" [suppressed]
move_body "Move1" [suppressed]
sketch "Sketch2" plane through (0, 0, 0) normal (0, 0, -1) x (-1, 0, 0)
  arc A0 (-500.0828, 983.0939) -> (-561.4783, 808.976) centre (-490.7581, 881.9227) ccw
  line L0 (-561.4783, 808.976) -> (-349.2633, 603.2383)
  arc A1 (-324.7055, 495.0118) -> (-349.2633, 603.2383) centre (-419.9835, 530.2916) ccw
  line L1 (-324.7055, 495.0118) -> (-508, 0)
  line L2 (-508, 0) -> (0, 0)
  line L3 (0, 0) -> (0, 1578.4878)
  arc A2 (0, 1578.4878) -> (-68.5744, 1674.5704) centre (-101.6, 1578.4878) ccw
  line L4 (-68.5744, 1674.5704) -> (-330.5174, 1764.6056)
  arc A3 (-330.5174, 1764.6056) -> (-463.7613, 1685.2216) centre (-363.543, 1668.5229) ccw
  arc A4 (-463.7613, 1685.2216) -> (-401.2067, 1607.5593) centre (-363.543, 1701.9203) ccw
  line L5 (-401.2067, 1607.5593) -> (-235.1219, 1541.2673)
  arc A5 (-176.4872, 1414.5155) -> (-235.1219, 1541.2673) centre (-272.7857, 1446.9063) ccw
  line L6 (-176.4872, 1414.5155) -> (-294.7966, 1062.7789)
  arc A6 (-381.7704, 993.9985) -> (-294.7966, 1062.7789) centre (-391.0951, 1095.1697) ccw
  line L7 (-381.7704, 993.9985) -> (-500.0828, 983.0939)
  line L8 (0, 0) -> (0, 1578.4878)
  constraint coincident L2.end L3.start
  constraint coincident L3.end A2.start
extrude "Extrude2" [suppressed]
sketch "Sketch3" plane through (0, 0, 0) normal (0, 0, -1) x (-1, 0, 0)
  arc A0 (-500.0828, 983.0939) -> (-561.4783, 808.976) centre (-490.7581, 881.9227) ccw
  line L0 (-561.4783, 808.976) -> (-349.2633, 603.2383)
  arc A1 (-324.7055, 495.0118) -> (-349.2633, 603.2383) centre (-419.9835, 530.2916) ccw
  line L1 (-324.7055, 495.0118) -> (-508, 0)
  line L2 (-508, 0) -> (0, 0)
  line L3 (0, 0) -> (0, 1578.4878)
  arc A2 (0, 1578.4878) -> (-68.5744, 1674.5704) centre (-101.6, 1578.4878) ccw
  line L4 (-68.5744, 1674.5704) -> (-330.5174, 1764.6056)
  arc A3 (-330.5174, 1764.6056) -> (-463.7613, 1685.2216) centre (-363.543, 1668.5229) ccw
  arc A4 (-463.7613, 1685.2216) -> (-401.2067, 1607.5593) centre (-363.543, 1701.9203) ccw
  line L5 (-401.2067, 1607.5593) -> (-235.1219, 1541.2673)
  arc A5 (-176.4872, 1414.5155) -> (-235.1219, 1541.2673) centre (-272.7857, 1446.9063) ccw
  line L6 (-176.4872, 1414.5155) -> (-294.7966, 1062.7789)
  arc A6 (-381.7704, 993.9985) -> (-294.7966, 1062.7789) centre (-391.0951, 1095.1697) ccw
  line L7 (-381.7704, 993.9985) -> (-500.0828, 983.0939)
  line L8 (-508, 0) -> (0, 0)
  constraint coincident L1.end L2.start
  constraint coincident L2.end L3.start
extrude "Extrude3" [suppressed]
sketch "Sketch4" plane through (0, 0, 0) normal (0, 0, -1) x (-1, 0, 0)
  arc A0 (-500.0828, 983.0939) -> (-561.4783, 808.976) centre (-490.7581, 881.9227) ccw
  line L0 (-561.4783, 808.976) -> (-349.2633, 603.2383)
  arc A1 (-324.7055, 495.0118) -> (-349.2633, 603.2383) centre (-419.9835, 530.2916) ccw
  line L1 (-324.7055, 495.0118) -> (-508, 0)
  line L2 (-508, 0) -> (0, 0)
  line L3 (0, 0) -> (0, 1578.4878)
  arc A2 (0, 1578.4878) -> (-68.5744, 1674.5704) centre (-101.6, 1578.4878) ccw
  line L4 (-68.5744, 1674.5704) -> (-330.5174, 1764.6056)
  arc A3 (-330.5174, 1764.6056) -> (-463.7613, 1685.2216) centre (-363.543, 1668.5229) ccw
  arc A4 (-463.7613, 1685.2216) -> (-401.2067, 1607.5593) centre (-363.543, 1701.9203) ccw
  line L5 (-401.2067, 1607.5593) -> (-235.1219, 1541.2673)
  arc A5 (-176.4872, 1414.5155) -> (-235.1219, 1541.2673) centre (-272.7857, 1446.9063) ccw
  line L6 (-176.4872, 1414.5155) -> (-294.7966, 1062.7789)
  arc A6 (-381.7704, 993.9985) -> (-294.7966, 1062.7789) centre (-391.0951, 1095.1697) ccw
  line L7 (-381.7704, 993.9985) -> (-500.0828, 983.0939)
  line L8 (-508, 0) -> (-375.4459, 357.9804)
  constraint coincident L1.end L2.start
  constraint parallel L1 L8
extrude "Extrude4" [suppressed]
move_body "Move2" [suppressed]
sketch "Sketch5" plane through (0, 0, 0) normal (0, 0, -1) x (-1, 0, 0)
  arc A0 (-500.0828, 983.0939) -> (-561.4783, 808.976) centre (-490.7581, 881.9227) ccw
  line L0 (-561.4783, 808.976) -> (-349.2633, 603.2383)
  arc A1 (-324.7055, 495.0118) -> (-349.2633, 603.2383) centre (-419.9835, 530.2916) ccw
  line L1 (-324.7055, 495.0118) -> (-508, 0)
  line L2 (-508, 0) -> (0, 0)
  line L3 (0, 0) -> (0, 1578.4878)
  arc A2 (0, 1578.4878) -> (-68.5744, 1674.5704) centre (-101.6, 1578.4878) ccw
  line L4 (-68.5744, 1674.5704) -> (-330.5174, 1764.6056)
  arc A3 (-330.5174, 1764.6056) -> (-463.7613, 1685.2216) centre (-363.543, 1668.5229) ccw
  arc A4 (-463.7613, 1685.2216) -> (-401.2067, 1607.5593) centre (-363.543, 1701.9203) ccw
  line L5 (-401.2067, 1607.5593) -> (-235.1219, 1541.2673)
  arc A5 (-176.4872, 1414.5155) -> (-235.1219, 1541.2673) centre (-272.7857, 1446.9063) ccw
  line L6 (-176.4872, 1414.5155) -> (-294.7966, 1062.7789)
  arc A6 (-381.7704, 993.9985) -> (-294.7966, 1062.7789) centre (-391.0951, 1095.1697) ccw
  line L7 (-381.7704, 993.9985) -> (-500.0828, 983.0939)
  line L8 (-561.7402, 704.8729) -> (-282.476, 272.5871)
extrude "Extrude5" [suppressed]
move_body "Move3" [suppressed]
extrude "Extrude6" [suppressed]
sketch "Sketch6" plane through (0, 0, 0) normal (0, 0, -1) x (-1, 0, 0)
  arc A0 (-500.0828, 983.0939) -> (-561.4783, 808.976) centre (-490.7581, 881.9227) ccw
  line L0 (-561.4783, 808.976) -> (-349.2633, 603.2383)
  arc A1 (-324.7055, 495.0118) -> (-349.2633, 603.2383) centre (-419.9835, 530.2916) ccw
  line L1 (-324.7055, 495.0118) -> (-508, 0)
  line L2 (-508, 0) -> (0, 0)
  line L3 (0, 0) -> (0, 1578.4878)
  arc A2 (0, 1578.4878) -> (-68.5744, 1674.5704) centre (-101.6, 1578.4878) ccw
  line L4 (-68.5744, 1674.5704) -> (-330.5174, 1764.6056)
  arc A3 (-330.5174, 1764.6056) -> (-463.7613, 1685.2216) centre (-363.543, 1668.5229) ccw
  arc A4 (-463.7613, 1685.2216) -> (-401.2067, 1607.5593) centre (-363.543, 1701.9203) ccw
  line L5 (-401.2067, 1607.5593) -> (-235.1219, 1541.2673)
  arc A5 (-176.4872, 1414.5155) -> (-235.1219, 1541.2673) centre (-272.7857, 1446.9063) ccw
  line L6 (-176.4872, 1414.5155) -> (-294.7966, 1062.7789)
  arc A6 (-381.7704, 993.9985) -> (-294.7966, 1062.7789) centre (-391.0951, 1095.1697) ccw
  line L7 (-381.7704, 993.9985) -> (-500.0828, 983.0939)
  line L8 (-535.57, 701.4712) -> (-535.57, 785.633)
  constraint vertical L8
extrude "Extrude7" [suppressed]
move_body "Move4" [suppressed]
sketch "Sketch7" plane through (0, 0, 0) normal (0, 0, -1) x (-1, 0, 0)
  arc A0 (-500.0828, 983.0939) -> (-561.4783, 808.976) centre (-490.7581, 881.9227) ccw
  line L0 (-561.4783, 808.976) -> (-349.2633, 603.2383)
  arc A1 (-324.7055, 495.0118) -> (-349.2633, 603.2383) centre (-419.9835, 530.2916) ccw
  line L1 (-324.7055, 495.0118) -> (-508, 0)
  line L2 (-508, 0) -> (0, 0)
  line L3 (0, 0) -> (0, 1578.4878)
  arc A2 (0, 1578.4878) -> (-68.5744, 1674.5704) centre (-101.6, 1578.4878) ccw
  line L4 (-68.5744, 1674.5704) -> (-330.5174, 1764.6056)
  arc A3 (-330.5174, 1764.6056) -> (-463.7613, 1685.2216) centre (-363.543, 1668.5229) ccw
  arc A4 (-463.7613, 1685.2216) -> (-401.2067, 1607.5593) centre (-363.543, 1701.9203) ccw
  line L5 (-401.2067, 1607.5593) -> (-235.1219, 1541.2673)
  arc A5 (-176.4872, 1414.5155) -> (-235.1219, 1541.2673) centre (-272.7857, 1446.9063) ccw
  line L6 (-176.4872, 1414.5155) -> (-294.7966, 1062.7789)
  arc A6 (-381.7704, 993.9985) -> (-294.7966, 1062.7789) centre (-391.0951, 1095.1697) ccw
  line L7 (-381.7704, 993.9985) -> (-500.0828, 983.0939)
  line L8 (-549.1372, 781.3002) -> (-199.0568, 871.2819)
extrude "Extrude8" [suppressed]
sketch "Sketch8" plane through (0, 0, 0) normal (0, 0, -1) x (-1, 0, 0)
  arc A0 (-500.0828, 983.0939) -> (-561.4783, 808.976) centre (-490.7581, 881.9227) ccw
  line L0 (-561.4783, 808.976) -> (-349.2633, 603.2383)
  arc A1 (-324.7055, 495.0118) -> (-349.2633, 603.2383) centre (-419.9835, 530.2916) ccw
  line L1 (-324.7055, 495.0118) -> (-508, 0)
  line L2 (-508, 0) -> (0, 0)
  line L3 (0, 0) -> (0, 1578.4878)
  arc A2 (0, 1578.4878) -> (-68.5744, 1674.5704) centre (-101.6, 1578.4878) ccw
  line L4 (-68.5744, 1674.5704) -> (-330.5174, 1764.6056)
  arc A3 (-330.5174, 1764.6056) -> (-463.7613, 1685.2216) centre (-363.543, 1668.5229) ccw
  arc A4 (-463.7613, 1685.2216) -> (-401.2067, 1607.5593) centre (-363.543, 1701.9203) ccw
  line L5 (-401.2067, 1607.5593) -> (-235.1219, 1541.2673)
  arc A5 (-176.4872, 1414.5155) -> (-235.1219, 1541.2673) centre (-272.7857, 1446.9063) ccw
  line L6 (-176.4872, 1414.5155) -> (-294.7966, 1062.7789)
  arc A6 (-381.7704, 993.9985) -> (-294.7966, 1062.7789) centre (-391.0951, 1095.1697) ccw
  line L7 (-381.7704, 993.9985) -> (-500.0828, 983.0939)
  line L8 (-209.0254, 871.1514) -> (-168.2196, 1302.162)
extrude "Extrude9" [suppressed]
sketch "Sketch9" plane through (0, 0, 0) normal (0, 0, -1) x (-1, 0, 0)
  arc A0 (-500.0828, 983.0939) -> (-561.4783, 808.976) centre (-490.7581, 881.9227) ccw
  line L0 (-561.4783, 808.976) -> (-349.2633, 603.2383)
  arc A1 (-324.7055, 495.0118) -> (-349.2633, 603.2383) centre (-419.9835, 530.2916) ccw
  line L1 (-324.7055, 495.0118) -> (-508, 0)
  line L2 (-508, 0) -> (0, 0)
  line L3 (0, 0) -> (0, 1578.4878)
  arc A2 (0, 1578.4878) -> (-68.5744, 1674.5704) centre (-101.6, 1578.4878) ccw
  line L4 (-68.5744, 1674.5704) -> (-330.5174, 1764.6056)
  arc A3 (-330.5174, 1764.6056) -> (-463.7613, 1685.2216) centre (-363.543, 1668.5229) ccw
  arc A4 (-463.7613, 1685.2216) -> (-401.2067, 1607.5593) centre (-363.543, 1701.9203) ccw
  line L5 (-401.2067, 1607.5593) -> (-235.1219, 1541.2673)
  arc A5 (-176.4872, 1414.5155) -> (-235.1219, 1541.2673) centre (-272.7857, 1446.9063) ccw
  line L6 (-176.4872, 1414.5155) -> (-294.7966, 1062.7789)
  arc A6 (-381.7704, 993.9985) -> (-294.7966, 1062.7789) centre (-391.0951, 1095.1697) ccw
  line L7 (-381.7704, 993.9985) -> (-500.0828, 983.0939)
  line L8 (-341.8169, 1393.1763) -> (-164.5669, 1284.7861)
extrude "Extrude10" [suppressed]
extrude "Extrude11" [suppressed]
sketch "Sketch11" plane through (0, 0, 0) normal (0, 0, -1) x (-1, 0, 0)
  line L0 (-354.0202, 344.3385) -> (-476.8204, 12.7)
  line L1 (-476.8204, 12.7) -> (0, 12.7)
  line L2 (0, 12.7) -> (0, 1578.4878)
  arc A0 (0, 1578.4878) -> (-68.5744, 1674.5704) centre (-101.6, 1578.4878) ccw
  line L3 (-68.5744, 1674.5704) -> (-330.5174, 1764.6056)
  arc A1 (-330.5174, 1764.6056) -> (-463.7613, 1685.2216) centre (-363.543, 1668.5229) ccw
  arc A2 (-463.7613, 1685.2216) -> (-401.2067, 1607.5593) centre (-363.543, 1701.9203) ccw
  line L4 (-401.2067, 1607.5593) -> (-235.1219, 1541.2673)
  arc A3 (-176.4872, 1414.5155) -> (-235.1219, 1541.2673) centre (-272.7857, 1446.9063) ccw
  line L5 (-176.4872, 1414.5155) -> (-294.7966, 1062.7789)
  arc A4 (-381.7704, 993.9985) -> (-294.7966, 1062.7789) centre (-391.0951, 1095.1697) ccw
  line L6 (-381.7704, 993.9985) -> (-500.0828, 983.0939)
  arc A5 (-500.0828, 983.0939) -> (-561.4783, 808.976) centre (-490.7581, 881.9227) ccw
  line L7 (-561.4783, 808.976) -> (-349.2633, 603.2383)
  arc A6 (-324.7055, 495.0118) -> (-349.2633, 603.2383) centre (-419.9835, 530.2916) ccw
  line L8 (-324.7055, 495.0118) -> (-508, 0)
  line L9 (-508, 0) -> (-481.523, 0)
  line L10 (-481.523, 0) -> (-477.7544, 10.1776)
  line L11 (-477.7544, 10.1776) -> (-489.6641, 14.5876)
  line L12 (-489.6641, 14.5876) -> (-365.93, 348.7485)
  line L13 (-365.93, 348.7485) -> (-354.0202, 344.3385)
  line L14 (-330.6788, 1500.205) -> (-330.6788, 1401.4151)
  constraint vertical L14
extrude "Extrude12" [suppressed]
sketch "Sketch12" plane through (0, 0, 0) normal (0, 0, -1) x (-1, 0, 0)
  line L0 (-354.0202, 344.3385) -> (-476.8204, 12.7)
  line L1 (-476.8204, 12.7) -> (0, 12.7)
  line L2 (0, 12.7) -> (0, 1578.4878)
  arc A0 (0, 1578.4878) -> (-68.5744, 1674.5704) centre (-101.6, 1578.4878) ccw
  line L3 (-68.5744, 1674.5704) -> (-330.5174, 1764.6056)
  arc A1 (-330.5174, 1764.6056) -> (-463.7613, 1685.2216) centre (-363.543, 1668.5229) ccw
  arc A2 (-463.7613, 1685.2216) -> (-401.2067, 1607.5593) centre (-363.543, 1701.9203) ccw
  line L4 (-401.2067, 1607.5593) -> (-235.1219, 1541.2673)
  arc A3 (-176.4872, 1414.5155) -> (-235.1219, 1541.2673) centre (-272.7857, 1446.9063) ccw
  line L5 (-176.4872, 1414.5155) -> (-294.7966, 1062.7789)
  arc A4 (-381.7704, 993.9985) -> (-294.7966, 1062.7789) centre (-391.0951, 1095.1697) ccw
  line L6 (-381.7704, 993.9985) -> (-500.0828, 983.0939)
  arc A5 (-500.0828, 983.0939) -> (-561.4783, 808.976) centre (-490.7581, 881.9227) ccw
  line L7 (-561.4783, 808.976) -> (-349.2633, 603.2383)
  arc A6 (-324.7055, 495.0118) -> (-349.2633, 603.2383) centre (-419.9835, 530.2916) ccw
  line L8 (-324.7055, 495.0118) -> (-508, 0)
  line L9 (-508, 0) -> (-481.523, 0)
  line L10 (-481.523, 0) -> (-477.7544, 10.1776)
  line L11 (-477.7544, 10.1776) -> (-489.6641, 14.5876)
  line L12 (-489.6641, 14.5876) -> (-365.93, 348.7485)
  line L13 (-365.93, 348.7485) -> (-354.0202, 344.3385)
  line L14 (-320.5243, 1498.2855) -> (-14.3023, 1396.529)
extrude "Extrude13" [suppressed]
extrude "Extrude14" [suppressed]
component "UpperShelf" placed x (1, 0, 0) y (0, 1, 0) z (0, 0, 1) at (0, 0, 0)
component "Bottom" placed x (1, 0, 0) y (0, 1, 0) z (0, 0, 1) at (0, 0, 0)
component "FrontConsole" placed x (1, 0, 0) y (0, 1, 0) z (0, 0, 1) at (0, 0, 0)
component "SideR Bottom" placed x (1, 0, 0) y (0, 1, 0) z (0, 0, 1) at (0, 0, 0)
component "BottomDoor" placed x (1, 0, 0) y (0, 1, 0) z (0, 0, 1) at (0, 0, 0)
component "Back Bottom" placed x (1, 0, 0) y (0, 1, 0) z (0, 0, 1) at (0, 0, 0)
component "SideLTop" placed x (1, 0, 0) y (0, 1, 0) z (0, 0, 1) at (0, 0, 0)
component "SideLBottom" placed x (1, 0, 0) y (0, 1, 0) z (0, 0, 1) at (0, 0, 0)
component "FrontLower" placed x (1, 0, 0) y (0, 1, 0) z (0, 0, 1) at (0, 0, 0)
component "SideR Top" placed x (1, 0, 0) y (0, 1, 0) z (0, 0, 1) at (0, 0, 0)
component "Screen" placed x (1, 0, 0) y (0, 1, 0) z (0, 0, 1) at (0, 0, 0)
component "Console" placed x (1, 0, 0) y (0, 1, 0) z (0, 0, 1) at (0, 0, 0)
component "Back Top" placed x (1, 0, 0) y (0, 1, 0) z (0, 0, 1) at (0, 0, 0)
component "LowerShelf" placed x (1, 0, 0) y (0, 1, 0) z (0, 0, 1) at (0, 0, 0)
component "Top" placed x (1, 0, 0) y (0, 1, 0) z (0, 0, 1) at (0, 0, 0)
component "FrontUpper" placed x (1, 0, 0) y (0, 1, 0) z (0, 0, 1) at (0, 0, 0)
component "TopDoor" placed x (1, 0, 0) y (0, 1, 0) z (0, 0, 1) at (0, 0, 0)
named bodies: "SideLBottom", "SideR Bottom", "Bottom", "Back Bottom", "FrontLower", "FrontUpper", "FrontConsole", "Console", "Screen", "Top", "SideLTop", "SideR Top", "UpperShelf", "Back Top", "LowerShelf", "TopDoor", "BottomDoor"
